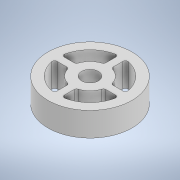
# Autodesk Inventor part: 6_10mm
Saved by Autodesk Inventor 2020 (Build 240168000, 168)
## iProperties
Created: 2021-02-20
Part Number: 6_10mm
Material: Generic
Document SubType Name: Modeling
Designer: Shuang Peng
Density: 1 g/cm^3
Appearance: Default
Author: Shuang Peng
Autodesk Inventor part; units mm, degrees
ref_plane "YZ Plane" through (0, 0, 0) normal (1, 0, 0) x (0, 1, 0)
ref_plane "XZ Plane" through (0, 0, 0) normal (0, 1, 0) x (-1, 0, 0)
ref_plane "XY Plane" through (0, 0, 0) normal (0, 0, 1) x (1, 0, 0)
sketch "Sketch1" plane through (0, 0, 0) normal (0, 1, 0) x (-1, 0, 0)
  circle A0 centre (0, 0) radius 3.5
  circle A1 centre (0, 0) radius 17.5
  circle A2 centre (0, 0) radius 7.5
  circle A3 centre (0, 0) radius 13.5
  line L0 (0, 0) -> (17.7641, 0)
  line L1 (15.8821, 1.5) -> (15.8821, -1.5)
  line L2 (15.8821, -1.5) -> (1.8821, -1.5)
  line L3 (1.8821, -1.5) -> (1.8821, 1.5)
  line L4 (1.8821, 1.5) -> (15.8821, 1.5)
  line L5 (15.8821, 1.5) -> (1.8821, -1.5) construction
  line L6 (15.8821, -1.5) -> (1.8821, 1.5) construction
  line L7 (0, 0) -> (8.8821, 0)
  line L8 (-1.5, -15.8821) -> (-1.5, -1.8821)
  line L9 (1.5, -1.8821) -> (1.5, -15.8821)
  line L10 (1.5, -15.8821) -> (-1.5, -15.8821)
  line L11 (-1.5, -1.8821) -> (1.5, -1.8821)
  line L12 (-15.8821, 1.5) -> (-1.8821, 1.5)
  line L13 (-1.8821, -1.5) -> (-15.8821, -1.5)
  line L14 (-15.8821, -1.5) -> (-15.8821, 1.5)
  line L15 (-1.8821, 1.5) -> (-1.8821, -1.5)
  line L16 (1.5, 15.8821) -> (1.5, 1.8821)
  line L17 (-1.5, 1.8821) -> (-1.5, 15.8821)
  line L18 (-1.5, 15.8821) -> (1.5, 15.8821)
  line L19 (1.5, 1.8821) -> (-1.5, 1.8821)
  point P0 (13.4164, -1.5)
  point P1 (1.5, -13.4164)
  point P2 (1.5, -7.3485)
  point P3 (7.3485, -1.5)
  point P4 (7.3485, 1.5)
  point P5 (1.5, 7.3485)
  point P6 (1.5, 13.4164)
  point P7 (13.4164, 1.5)
  point P8 (-1.5, -7.3485)
  point P9 (-1.5, -13.4164)
  point P10 (-13.4164, -1.5)
  point P11 (-7.3485, -1.5)
  point P12 (-7.3485, 1.5)
  point P13 (-13.4164, 1.5)
  point P14 (-1.5, 13.4164)
  point P15 (-1.5, 7.3485)
  dimension "d0" = 7
  dimension "d1" = 35
  dimension "d2" = 4
  dimension "d3" = 4
  dimension "d4" = 3
  dimension "d5" = 14
  dimension "d8" = 360
  constraints: 40 end point, 6 coincident, 4 centre point, 3 midpoint, 2 parallel, 2 perpendicular, 1 collinear, 1 horizontal, 35 other
  measures "d0" diameter of A0
  measures "d1" diameter of A1
  measures "d2" radial gap between concentric circles of A0 A2
  measures "d3" radial gap between concentric circles of A1 A3
  measures "d4" distance of L1.start L1.end
  measures "d5" distance of L1.end L2.end
extrude "Extrusion1" add sketch "Sketch1" along normal blind 10 contours L0 A2 L2 A0 | A0 L4 A2 L0 | A0 L16 A2 L4 | L2 A2 L9 A0 | L0 A3 L2 A2 | A2 L4 A3 L0 | A0 L17 A2 L16 | L9 A2 L8 A0 | A0 L12 A2 L17 | A2 L17 A3 L16 | L4 L1 L0 A3 | A1 | L8 A2 L13 A0 | L9 A3 L8 A2 | A3 L0 L1 L2 | A0 L13 A2 L12 | A3 L17 L18 L16 | L9 L10 L8 A3 | A2 L13 A3 L12 | A3 L13 L14 L12
fillet "Fillet1" radius 1 16 edges at (13.4164, 5, -1.5) (1.5, 5, -13.4164) (1.5, 5, -7.3485) (-1.5, 5, -7.3485) (7.3485, 5, -1.5) (-7.3485, 5, -1.5) (-7.3485, 5, 1.5) (-1.5, 5, 7.3485) (1.5, 5, 7.3485) (7.3485, 5, 1.5) (13.4164, 5, 1.5) (1.5, 5, 13.4164) (-1.5, 5, 13.4164) (-13.4164, 5, 1.5) (-13.4164, 5, -1.5) (-1.5, 5, -13.4164)
body "Solid1"
